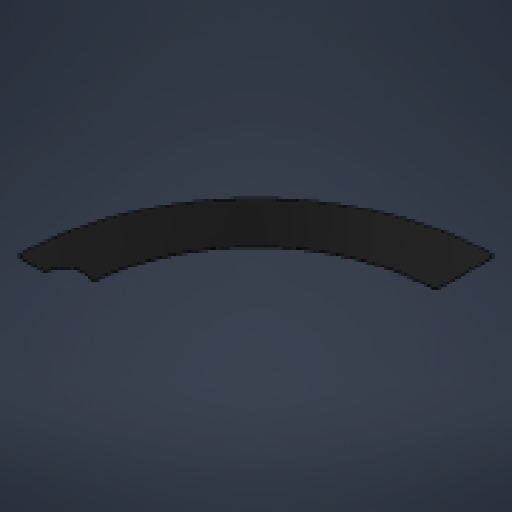
# Autodesk Inventor part: 3DPRINT,CABLE,GUARD
Saved by Autodesk Inventor 2026.1 (Build 301233020, 233B)
## iProperties
Created: 2026-02-15
Part Number: 3DPRINT,CABLE,GUARD
Material: ABS Plastic
Document SubType Name: Modeling
Designer: Owen L
Density: 1.06 g/cm^3
Appearance: Smooth - Black
Author: Owen L
Autodesk Inventor part; units mm, degrees
ref_plane "YZ Plane" through (0, 0, 0) normal (1, 0, 0) x (0, 1, 0)
ref_plane "XZ Plane" through (0, 0, 0) normal (0, 1, 0) x (-1, 0, 0)
ref_plane "XY Plane" through (0, 0, 0) normal (0, 0, 1) x (1, 0, 0)
sketch "Sketch1" plane through (0, 0, 0) normal (0, 1, 0) x (-1, 0, 0)
  arc A0 (0, -179.3875) -> (179.3875, 0) centre (0, 0) ccw
  arc A1 (0, -134.9375) -> (134.9375, 0) centre (0, 0) ccw
  line L0 (179.3875, 0) -> (134.9375, 0)
  line L1 (0, -134.9375) -> (0, -179.3875)
  point P0 (0, -157.1625)
  point P1 (157.1625, 0)
  dimension "d0" = 179.3875
  dimension "d1" = 134.9375
  constraints: 4 end point, 4 point on circle, 2 centre point, 2 coincident, 2 midpoint, 1 horizontal, 1 horizontal alignment, 1 perpendicular, 1 vertical alignment
  measures "d0" radius of A0
  measures "d1" radius of A1
extrude "Extrusion1" add sketch "Sketch1" along normal blind 0.4
sketch "Sketch2" plane through (0, 0.4, 0) normal (0, 1, 0) x (1, 0, 0)
  line L0 (-179.3875, 0) -> (-134.9375, 0) projected
  circle A0 centre (-143.51, 0) radius 14.2875
  point P0 (0, 0)
  dimension "d4" = 143.51
  dimension "d5" = 28.575
  constraints: 1 centre point, 1 point on line
  measures "d4" distance of point (0, 0) A0.centre
  measures "d5" diameter of A0
extrude "Extrusion2" cut sketch "Sketch2" against normal through all
fillet "Fillet1" radius 1.5875 5 edges at (-134.4823, 0.2, -11.074) (-157.7975, 0.2, 0) (-179.3875, 0.2, 0) (0, 0.2, -134.9375) (0, 0.2, -179.3875)
body "Solid1"
